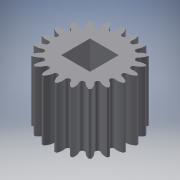
# Autodesk Inventor part: gear 4 shaft
Saved by Autodesk Inventor 2017 (Build 210142000, 142)
## iProperties
Created: 2018-04-17
Part Number: gear 4 shaft
Material: Generic
Document SubType Name: Modeling
Designer: RKL
Density: 1 g/cm^3
Appearance: Default
Author: RKL
Autodesk Inventor part; units mm, degrees
ref_plane "YZ Plane" through (0, 0, 0) normal (1, 0, 0) x (0, 1, 0)
ref_plane "XZ Plane" through (0, 0, 0) normal (0, 1, 0) x (-1, 0, 0)
ref_plane "XY Plane" through (0, 0, 0) normal (0, 0, 1) x (1, 0, 0)
sketch "Sketch1" plane through (0, 0, 0) normal (0, 0, 1) x (1, 0, 0)
  spline S0 degree 3 poles (-1.8349, 13.6245) (-1.724, 13.4816) (-1.5022, 13.1956) (-1.2174, 12.7324) (-1.0219, 12.3241) (-0.8975, 11.9834) (-0.8637, 11.8055) (-0.8468, 11.7167) knots 0 0 0 0 0.054257 0.10851 0.162749 0.189878 0.21698 0.21698 0.21698 0.21698
  spline S1 degree 3 poles (-0.8468, 11.7167) (-0.8343, 11.5885) (-0.8156, 11.3963) (-0.7404, 11.1497) (-0.6556, 10.9758) (-0.5351, 10.8232) (-0.3789, 10.7074) (-0.1935, 10.6418) (0, 10.6468) (0.1935, 10.6418) (0.3789, 10.7074) (0.5351, 10.8232) (0.6556, 10.9758) (0.7404, 11.1497) (0.8156, 11.3963) (0.8343, 11.5885) (0.8468, 11.7167) knots 0 0 0 0 0.038496 0.057749 0.077012 0.096258 0.11548 0.134682 0.153929 0.173175 0.192377 0.2116 0.230846 0.250109 0.269362 0.307858 0.307858 0.307858 0.307858
  spline S2 degree 3 poles (0.8468, 11.7167) (0.8637, 11.8055) (0.8975, 11.9834) (1.0219, 12.3241) (1.2174, 12.7324) (1.5022, 13.1956) (1.724, 13.4816) (1.8349, 13.6245) knots 0 0 0 0 0.027102 0.05423 0.10847 0.162723 0.21698 0.21698 0.21698 0.21698
  circle A0 centre (0, 0) radius 10.6451 construction
  circle A1 centre (0, 0) radius 11.7462 construction
  circle A2 centre (0, 0) radius 12.5 construction
  circle A3 centre (0, 0) radius 13.7475
  point P0 (-1.5102, 13.1899)
  point P1 (-1.2257, 12.7279)
  point P2 (-0.9935, 12.2377)
  point P3 (-0.9046, 11.9814)
  point P4 (-0.7926, 11.3355)
  point P5 (-0.7357, 11.1516)
  point P6 (-0.6496, 10.9793)
  point P7 (-0.5291, 10.8292)
  point P8 (-0.374, 10.7157)
  point P9 (-0.1923, 10.6536)
  point P10 (0, 10.6451)
  point P11 (0.1923, 10.6536)
  point P12 (0.374, 10.7157)
  point P13 (0.5291, 10.8292)
  point P14 (0.6496, 10.9793)
  point P15 (0.7357, 11.1516)
  point P16 (0.7926, 11.3355)
  point P17 (0.9046, 11.9814)
  point P18 (0.9935, 12.2377)
  point P19 (1.2257, 12.7279)
  point P20 (1.5102, 13.1899)
  constraints: 4 centre point, 2 point on circle, 57 other
extrude "Extrusion1" add sketch "Sketch1" against normal blind 20
extrude "Extrusion2" cut sketch "Sketch1" against normal through all contours A3 S2 S1 S0 picked at (0.1949, 12.7504)
pattern_circular "Circular Pattern1" count 20 over 360 about axis through (0, 0, 0) along (0, 0, -1) of "Extrusion2"
sketch "Sketch2" plane through (0, 0, 0) normal (0, 0, 1) x (1, 0, 0)
  line L0 (4.7625, -4.7625) -> (-4.7625, -4.7625)
  line L1 (-4.7625, -4.7625) -> (-4.7625, 4.7625)
  line L2 (-4.7625, 4.7625) -> (4.7625, 4.7625)
  line L3 (4.7625, 4.7625) -> (4.7625, -4.7625)
  line L4 (4.7625, -4.7625) -> (-4.7625, 4.7625) construction
  line L5 (-4.7625, -4.7625) -> (4.7625, 4.7625) construction
  point P0 (0, 0)
  dimension "d7" = 9.525
  constraints: 12 end point, 2 midpoint, 2 parallel, 2 perpendicular, 1 horizontal
  measures "d7" distance of L0.end L1.end
extrude "Extrusion3" cut sketch "Sketch2" against normal through all
equation "\"d0\" = FaceWidth"
equation "\"Module\" = 1.25"
equation "\"PressureAngle\" = 20deg"
equation "\"UnitProfileClearance\" = 0.25"
equation "\"UnitRoundRadius\" = 0.35"
equation "\"HeadDiameter\" = 27.49508"
equation "\"RootDiameter\" = 21.29024"
equation "\"BaseDiameter\" = 23.49232"
equation "\"PitchDiameter\" = 25"
equation "\"FaceWidth\" = 20"
equation "\"HelixAngle\" = 0"
equation "\"UnitCorrection\" = 0"
equation "\"UnitAddendumModification\" = 0.001969"
equation "\"CircularPitch\" = 3.926991"
equation "\"UnitBacklashShift\" = -0.233904"
equation "\"TotalToolShift\" = -0.29238"
equation "\"IsInternal\" = 0"
body "Solid1"
